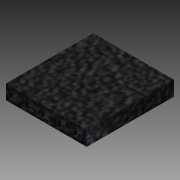
# Autodesk Inventor part: Five Pin Plug
Saved by Autodesk Inventor 2014 (Build 180170000, 170)
## iProperties
Created: 2014-02-26
Part Number: Five Pin Plug
Material: Generic
Document SubType Name: Modeling
Designer: Spooner
Density: 1 g/cm^3
Appearance: Black Cast
Author: Spooner
Autodesk Inventor part; units mm, degrees
ref_plane "YZ Plane" through (0, 0, 0) normal (1, 0, 0) x (0, 1, 0)
ref_plane "XZ Plane" through (0, 0, 0) normal (0, 1, 0) x (-1, 0, 0)
ref_plane "XY Plane" through (0, 0, 0) normal (0, 0, 1) x (1, 0, 0)
sketch "Sketch1" plane through (0, 0, 0) normal (0, 1, 0) x (-1, 0, 0)
  line L0 (0, 0) -> (12.7, 0)
  line L1 (12.7, 0) -> (12.7, 13.716)
  line L2 (12.7, 13.716) -> (0, 13.716)
  line L3 (0, 13.716) -> (0, 0)
  dimension "d0" = 12.7
  dimension "d1" = 13.716
  constraints: 8 end point, 2 parallel, 1 horizontal, 1 perpendicular
  measures "d0" distance of L0.start L0.end
  measures "d1" distance of L2.end L0.start
extrude "Extrusion1" add sketch "Sketch1" along normal blind 2.286
sketch "Sketch2" plane through (-12.7, 0, 13.716) normal (0, 0, 1) x (1, 0, 0)
  line L0 (0, 2.286) -> (12.7, 2.286) projected
  line L1 (0, 0) -> (0, 2.286) projected
  line L2 (0.762, 1.524) -> (1.524, 1.524)
  line L3 (1.524, 1.524) -> (1.524, 0.762)
  line L4 (1.524, 0.762) -> (0.762, 0.762)
  line L5 (0.762, 0.762) -> (0.762, 1.524)
  dimension "d4" = 0.762
  dimension "d5" = 0.762
  dimension "d6" = 0.762
  dimension "d7" = 0.762
  constraints: 8 end point, 2 parallel, 1 horizontal, 1 perpendicular
  measures "d4" distance of L2.start L2.end
  measures "d5" distance of L4.end L2.start
  measures "d6" distance between parallel lines of L0 L2
  measures "d7" distance between parallel lines of L1 L5
extrude "Extrusion2" cut sketch "Sketch2" against normal blind 12.7
chamfer "Chamfer1" distance 0.254 angle 45 4 edges at (-11.938, 1.143, 13.716) (-11.557, 1.524, 13.716) (-11.176, 1.143, 13.716) (-11.557, 0.762, 13.716)
sketch "Sketch3" plane through (0, 0, 0) normal (0, 0, -1) x (-1, 0, 0)
  line L0 (11.938, 1.524) -> (11.176, 1.524) projected
  line L1 (11.938, 0.762) -> (11.938, 1.524) projected
  line L2 (11.176, 0.762) -> (11.938, 0.762) projected
  line L3 (11.176, 1.524) -> (11.176, 0.762) projected
  circle A0 centre (11.557, 1.143) radius 0.2335
  point P0 (11.557, 1.524)
  point P1 (11.176, 1.143)
  constraints: 2 midpoint, 1 centre point, 1 horizontal alignment, 1 vertical alignment
extrude "Extrusion3" cut sketch "Sketch3" against normal blind 0.6477 contours A0
sketch "Sketch4" plane through (0, 0, 0) normal (0, -1, 0) x (1, 0, 0)
  line L0 (-12.7, 13.716) -> (0, 13.716) projected
  line L1 (-12.7, 0) -> (-12.7, 13.716) projected
  line L2 (-11.176, 13.462) -> (-11.176, 1.016) projected
  line L3 (-11.938, 13.462) -> (-11.938, 1.016) projected
  line L4 (-11.176, 1.016) -> (-11.938, 1.016) projected
  line L5 (-12.192, 9.906) -> (-10.922, 9.906)
  line L6 (-10.922, 9.906) -> (-10.922, 8.636)
  line L7 (-10.922, 8.636) -> (-12.192, 8.636)
  line L8 (-12.192, 8.636) -> (-12.192, 9.906)
  dimension "d18" = 0.508
  dimension "d19" = 1.27
  dimension "d20" = 1.27
  dimension "d21" = 3.81
  constraints: 8 end point, 2 parallel, 1 horizontal, 1 perpendicular
  measures "d18" distance between parallel lines of L1 L8
  measures "d19" distance of L6.end L7.end
  measures "d20" distance of L5.end L6.end
  measures "d21" distance between parallel lines of L0 L5
extrude "Extrusion4" cut sketch "Sketch4" against normal blind 0.127 contours L5 L6 L7 L2 | L2 L7 L3 L5 | L3 L7 L8 L5
pattern_linear "Rectangular Pattern1" count 5 spacing 2.54 along (1, 0, 0) of "Extrusion2", "Chamfer1", "Extrusion3", "Extrusion4"
body "Solid1"
